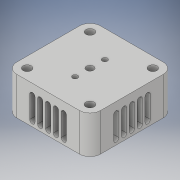
# Autodesk Inventor part: Air Zone
Saved by Autodesk Inventor 2018 (Build 220112000, 112)
## iProperties
Created: 2020-03-23
Part Number: Air Zone
Material: Generic
Document SubType Name: Modeling
Designer: emile
Density: 1 g/cm^3
Appearance: Default
Author: emile
Autodesk Inventor part; units mm, degrees
ref_plane "YZ Plane" through (0, 0, 0) normal (1, 0, 0) x (0, 1, 0)
ref_plane "XZ Plane" through (0, 0, 0) normal (0, 1, 0) x (-1, 0, 0)
ref_plane "XY Plane" through (0, 0, 0) normal (0, 0, 1) x (1, 0, 0)
sketch "Sketch1" plane through (0, 0, 0) normal (0, 1, 0) x (-1, 0, 0)
  circle A0 centre (0, 0) radius 42.2275
  circle A1 centre (0, 0) radius 50.8
  line L0 (0, 50.8) -> (-50.8, 50.8)
  line L1 (-50.8, 50.8) -> (-50.8, -50.8)
  line L2 (-50.8, -50.8) -> (0, -50.8)
  circle A2 centre (0, 0) radius 39.0525
  circle A3 centre (0, 0) radius 35.8775
  circle A4 centre (0, 0) radius 32.7025
  circle A5 centre (0, 0) radius 29.5275
  circle A6 centre (0, 0) radius 26.3525
  circle A7 centre (0, 0) radius 23.1775
  circle A8 centre (0, 0) radius 20.0025
  circle A9 centre (0, 0) radius 16.8275
  circle A10 centre (0, 0) radius 13.6525
  circle A11 centre (0, 0) radius 10.4775
  line L3 (0, 3.175) -> (42.2275, 3.175)
  line L4 (42.2275, 3.175) -> (42.2275, -3.175)
  line L5 (42.2275, -3.175) -> (0, -3.175)
  line L6 (0, -3.175) -> (0, 3.175)
  line L7 (0, -50.8) -> (50.8, -50.8)
  line L8 (50.8, -50.8) -> (50.8, 0)
  point P0 (42.2275, 0)
  dimension "d0" = 84.455
  dimension "d2" = 50.8
  dimension "d3" = 50.8
  dimension "d6" = 3.175
  dimension "d7" = 3.175
  dimension "d8" = 3.175
  dimension "d9" = 3.175
  dimension "d10" = 3.175
  dimension "d11" = 3.175
  dimension "d12" = 3.175
  dimension "d13" = 3.175
  dimension "d14" = 3.175
  dimension "d15" = 3.175
  dimension "d16" = 6.35
  constraints: 18 end point, 13 coincident, 11 centre point, 4 perpendicular, 4 tangent, 3 point on circle, 2 horizontal, 2 midpoint, 2 parallel, 1 horizontal alignment, 2 other
  measures "d2" distance from line of L0 point (0, 0)
  measures "d3" distance from line of point (0, 0) L2
  measures "d7" radial gap between concentric circles of A2 A3
  measures "d8" radial gap between concentric circles of A3 A4
  measures "d9" radial gap between concentric circles of A4 A5
  measures "d10" radial gap between concentric circles of A5 A6
  measures "d11" radial gap between concentric circles of A6 A7
  measures "d12" radial gap between concentric circles of A7 A8
  measures "d13" radial gap between concentric circles of A8 A9
  measures "d14" radial gap between concentric circles of A9 A10
  measures "d15" radial gap between concentric circles of A10 A11
  measures "d16" distance between parallel lines of L5 L3
extrude "Extrusion1" add sketch "Sketch1" along normal blind 45.7708 contours A1 | A1 L1 L0 | L2 L1 A1
sketch "Sketch4" plane through (0, 45.7708, 0) normal (0, 1, 0) x (1, 0, 0)
  line L0 (0, -50.8) -> (50.8, -50.8) projected
  line L1 (50.8, -50.8) -> (50.8, 50.8) projected
  line L2 (50.8, 50.8) -> (0, 50.8) projected
  arc A0 (0, 50.8) -> (0, -50.8) centre (0, 0) ccw projected
  arc A1 (-42.108, -3.175) -> (-42.108, 3.175) centre (0, 0) ccw projected
  line L3 (-42.108, -3.175) -> (-42.2275, -3.175) projected
  line L4 (-42.2275, -3.175) -> (-42.2275, 3.175) projected
  line L5 (-42.2275, 3.175) -> (-42.108, 3.175) projected
sketch "Sketch7" plane through (0, 45.7708, 0) normal (0, 1, 0) x (1, 0, 0)
  point P0 (0, 0)
extrude "Extrusion13" add sketch "Sketch1" along normal up to surface (45.7708 mm away) contours L8 L7 A1
sketch "Sketch13" plane through (0, 45.7708, 0) normal (0, 1, 0) x (1, 0, 0)
  line L0 (0, -50.8) -> (50.8, -50.8) projected
  line L1 (50.8, -50.8) -> (50.8, 50.8) projected
  line L2 (50.8, 50.8) -> (-50.8, 50.8) projected
  line L3 (-50.8, 0) -> (-50.8, 50.8) projected
  arc A0 (-50.8, 0) -> (0, -50.8) centre (0, 0) ccw projected
  arc A1 (-42.108, -3.175) -> (-42.108, 3.175) centre (0, 0) ccw projected
  line L4 (-42.108, -3.175) -> (-42.2275, -3.175) projected
  line L5 (-42.2275, -3.175) -> (-42.2275, 3.175) projected
  line L6 (-42.2275, 3.175) -> (-42.108, 3.175) projected
  line L7 (-42.2275, 3.175) -> (-42.108, 3.175) projected
  circle A2 centre (0, 0) radius 42.2275
  constraints: 1 coincident, 3 other
extrude "Extrusion14" add sketch "Sketch13" against normal up to surface (45.7708 mm away) contours L4 L5 A2 | L5 L6 A2
sketch "Sketch14" plane through (0, 45.7708, 0) normal (0, 1, 0) x (1, 0, 0)
  line L0 (0, -50.8) -> (50.8, -50.8) projected
  line L1 (50.8, -50.8) -> (50.8, 50.8) projected
  line L2 (50.8, 50.8) -> (-50.8, 50.8) projected
  line L3 (-50.8, 0) -> (-50.8, 50.8) projected
  arc A0 (-50.8, 0) -> (0, -50.8) centre (0, 0) ccw projected
  circle A1 centre (0, 0) radius 42.2275 projected
extrude "Extrusion15" add sketch "Sketch14" against normal blind 9.525 contours A1
sketch "Sketch15" plane through (0, 45.7708, 0) normal (0, 1, 0) x (1, 0, 0)
  circle A0 centre (0, -18) radius 3.175
  circle A1 centre (0, 18) radius 3.175
  circle A2 centre (0, 0) radius 4.3656
  circle A3 centre (-38.1, 38.1) radius 5.0419
  circle A4 centre (38.1, 38.1) radius 5.0419
  circle A5 centre (38.1, -38.1) radius 5.0419
  line L0 (-50.8, 0) -> (-50.8, 50.8) projected
  line L1 (50.8, 50.8) -> (-50.8, 50.8) projected
  line L2 (50.8, -50.8) -> (50.8, 50.8) projected
  line L3 (0, -50.8) -> (50.8, -50.8) projected
  dimension "d57" = 8.7312
  dimension "d58" = 36
  dimension "d59" = 18
  dimension "d60" = 6.35
  dimension "d63" = 10.0838
  dimension "d64" = 12.7
  dimension "d65" = 12.7
  dimension "d66" = 12.7
  dimension "d67" = 12.7
  constraints: 6 centre point, 3 equal radius, 3 vertical alignment, 1 coincident, 1 horizontal alignment
  measures "d57" diameter of A2
  measures "d58" distance of A0.centre A1.centre
  measures "d59" distance of A0.centre A2.centre
  measures "d60" diameter of A1
  measures "d63" diameter of A3
  measures "d64" distance from line of L0 A3.centre
  measures "d65" distance from line of L1 A3.centre
  measures "d66" distance from line of L2 A4.centre
  measures "d67" distance from line of L3 A5.centre
extrude "Extrusion16" cut sketch "Sketch15" against normal through all contours A0 | A1 | A2
extrude "Extrusion17" cut sketch "Sketch15" against normal through all contours A3 | A4 | A5
sketch "Sketch19" plane through (50.8, 0, 50.8) normal (1, 0, 0) x (0, 0, -1)
  point P0 (50.8, 0)
sketch "Sketch20" plane through (50.8, 0, -50.8) normal (0, 0, -1) x (-1, 0, 0)
  line L0 (0, 0) -> (101.6, 0) projected
  line L1 (101.6, 0) -> (101.6, 45.7708) projected
  line L2 (0, 45.7708) -> (101.6, 45.7708) projected
  line L3 (0, 0) -> (0, 45.7708) projected
  line L4 (93.0275, 36.2458) -> (8.5725, 36.2458) projected
  line L5 (50.8, 0) -> (50.8, 45.7708) projected
  line L6 (50.8, 6.35) -> (50.8, 33.0708) construction
  line L7 (53.975, 36.2458) -> (47.625, 36.2458) projected
  line L8 (47.625, 6.35) -> (47.625, 33.0708)
  line L9 (53.975, 33.0708) -> (53.975, 6.35)
  arc A0 (47.625, 6.35) -> (53.975, 6.35) centre (50.8, 6.35) ccw
  arc A1 (53.975, 33.0708) -> (47.625, 33.0708) centre (50.8, 33.0708) ccw
  point P0 (50.8, 19.7104)
  dimension "d95" = 6.35
  dimension "d96" = 6.35
  constraints: 8 end point, 5 tangent, 4 point on circle, 2 centre point, 1 midpoint, 1 parallel, 1 perpendicular, 1 point on line
  measures "d95" distance from line of L0 L6.start
  measures "d96" distance between parallel lines of L8 L9
extrude "Extrusion21" cut sketch "Sketch20" against normal blind 43.5102 contours A0 L8 A1 L5 | L5 A1 L9 A0
pattern_linear "Rectangular Pattern1" count 3 spacing 9.525 along (-1, 0, 0) of "Extrusion21"
mirror "Mirror1" about plane through (0, 0, 0) normal (1, 0, 0) of "Extrusion21", "Rectangular Pattern1"
sketch "Sketch21" plane through (0, 0, 0) normal (0, -1, 0) x (1, 0, 0)
  circle A0 centre (38.1, -38.1) radius 5.0419 projected
  circle A1 centre (-38.1, -38.1) radius 5.0419 projected
  circle A2 centre (38.1, 38.1) radius 5.0419 projected
  circle A3 centre (0, 0) radius 42.2275 projected
  line L0 (0, 50.8) -> (50.8, 50.8) projected
  arc A4 (0, 50.8) -> (-50.8, 0) centre (0, 0) ccw projected
  line L1 (-50.8, -50.8) -> (-50.8, 0) projected
  line L2 (50.8, -50.8) -> (-50.8, -50.8) projected
  line L3 (50.8, 50.8) -> (50.8, -50.8) projected
  arc A5 (0, 50.8) -> (-50.8, 0) centre (0, 0) ccw projected
  line L4 (0, 50.8) -> (-50.8, 50.8)
  line L5 (0, 50.8) -> (50.8, 50.8) projected
  line L6 (-50.8, 50.8) -> (0, 50.8)
  line L7 (-50.8, 0) -> (-50.8, -50.8) projected
  line L8 (-50.8, 50.8) -> (-50.8, 0)
  circle A6 centre (-38.1, 38.1) radius 5.0419
  circle A7 centre (-38.1, -38.1) radius 5.0419 projected
  arc A8 (0, 50.8) -> (-50.8, 0) centre (0, 0) ccw projected
  constraints: 6 end point, 2 collinear, 2 tangent, 1 centre point, 1 equal radius, 1 horizontal alignment, 1 vertical alignment
extrude "Extrusion22" add sketch "Sketch21" against normal up to surface (45.7708 mm away) contours A4 A6 L8 L4 | A4 A6 picked at (-37.6782, 37.9609)
extrude "Extrusion23" cut sketch "Sketch21" against normal through all contours A6 A4 | A4 A6
fillet "Fillet2" radius 12.7 4 edges at (50.8, 22.8854, 50.8) (-50.8, 22.8854, 50.8) (-50.8, 22.8854, -50.8) (50.8, 22.8854, -50.8)
pattern_circular "Circular Pattern3" count 4 over 360 about axis through (0, 0, 0) along (0, 1, 0) of "Extrusion21", "Rectangular Pattern1", "Mirror1"
ref_plane "Work Plane1" through (0, 0, 0) normal (1, 0, 0) x (0, 1, 0)
ref_plane "Work Plane2" through (0, 0, 0) normal (0, 0, -1) x (0, 1, 0)
ref_plane "Work Plane3" through (0, 0, 0) normal (-1, 0, 0) x (0, 1, 0)
ref_plane "Work Plane4" through (0, 0, 0) normal (0, 0, 1) x (0, 1, 0)
ref_plane "Work Plane5" through (0, 0, 0) normal (0, 0, -1) x (0, 1, 0)
ref_plane "Work Plane6" through (0, 0, 0) normal (-1, 0, 0) x (0, 1, 0)
ref_plane "Work Plane7" through (0, 0, 0) normal (0, 0, 1) x (0, 1, 0)
equation "\"d3\" = d2"
equation "\"d8\" = d7"
equation "\"d9\" = d8"
equation "\"d10\" = d9"
equation "\"d11\" = d10"
equation "\"d12\" = d11"
equation "\"d13\" = d10"
equation "\"d14\" = d13"
equation "\"d15\" = d13"
equation "\"d59\" = 0.5 * d58"
equation "\"d65\" = d64"
equation "\"d66\" = d64"
equation "\"d67\" = d66"
body "Solid1"
